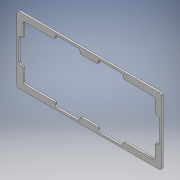
# Autodesk Inventor part: layer3
Saved by Autodesk Inventor 2017 (Build 210142000, 142)
## iProperties
Created: 2021-06-16
Part Number: layer3
Material: Generic
Document SubType Name: Modeling
Designer: Jack
Density: 1 g/cm^3
Appearance: Default
Author: Jack
Autodesk Inventor part; units mm, degrees
ref_plane "YZ Plane" through (0, 0, 0) normal (1, 0, 0) x (0, 1, 0)
ref_plane "XZ Plane" through (0, 0, 0) normal (0, 1, 0) x (-1, 0, 0)
ref_plane "XY Plane" through (0, 0, 0) normal (0, 0, 1) x (1, 0, 0)
sketch "Sketch1" plane through (0, 0, 0) normal (0, 1, 0) x (-1, 0, 0)
  line L0 (-161.0144, 75.423) -> (-161.0144, -74.402)
  line L1 (-156.0144, 80.423) -> (179.5486, 80.423)
  arc A0 (-156.0144, 80.423) -> (-161.0144, 75.423) centre (-156.0144, 75.423) ccw
  arc A1 (-161.0144, -74.402) -> (-156.0144, -79.402) centre (-156.0144, -74.402) ccw
  line L2 (184.5486, -74.402) -> (184.5486, 75.423)
  line L3 (179.5486, -79.402) -> (-156.0144, -79.402)
  arc A2 (179.5486, -79.402) -> (184.5486, -74.402) centre (179.5486, -74.402) ccw
  arc A3 (184.5486, 75.423) -> (179.5486, 80.423) centre (179.5486, 75.423) ccw
  line L4 (-143.0264, 65.4235) -> (-72.3404, 65.4235)
  line L5 (169.5485, 62.4233) -> (169.5485, 33.0083)
  line L6 (-146.0144, -61.402) -> (-146.0144, -31.9917)
  line L7 (-146.0144, 62.4233) -> (-146.0144, 33.0083)
  line L8 (-156.0144, 0.5083) -> (-156.0144, -24.4917)
  line L9 (-156.0144, 0.5083) -> (-156.0144, 25.5083)
  line L10 (-151.0144, -29.4917) -> (-148.5144, -29.4917)
  line L11 (-151.0144, 30.5083) -> (-148.5144, 30.5083)
  line L12 (-7.3404, 65.4235) -> (30.8506, 65.4235)
  line L13 (166.5366, 65.4235) -> (95.8506, 65.4235)
  arc A4 (-151.0144, 30.5083) -> (-156.0144, 25.5083) centre (-151.0144, 25.5083) ccw
  arc A5 (-156.0144, -24.4917) -> (-151.0144, -29.4917) centre (-151.0144, -24.4917) ccw
  arc A6 (-146.0144, -31.9917) -> (-148.5144, -29.4917) centre (-148.5144, -31.9917) ccw
  arc A7 (-148.5144, 30.5083) -> (-146.0144, 33.0083) centre (-148.5144, 33.0083) ccw
  line L14 (179.5485, 0.5083) -> (179.5485, 25.5083)
  line L15 (179.5485, 0.5083) -> (179.5485, -24.4917)
  line L16 (174.5485, 30.5083) -> (172.0485, 30.5083)
  line L17 (174.5485, -29.4917) -> (172.0485, -29.4917)
  arc A8 (174.5485, -29.4917) -> (179.5485, -24.4917) centre (174.5485, -24.4917) ccw
  arc A9 (179.5485, 25.5083) -> (174.5485, 30.5083) centre (174.5485, 25.5083) ccw
  arc A10 (169.5485, 33.0083) -> (172.0485, 30.5083) centre (172.0485, 33.0083) ccw
  arc A11 (172.0485, -29.4917) -> (169.5485, -31.9917) centre (172.0485, -31.9917) ccw
  line L18 (169.5485, -31.9917) -> (169.5485, -61.402)
  line L19 (-39.8404, 75.4235) -> (-64.8404, 75.4235)
  line L20 (-39.8404, 75.4235) -> (-14.8404, 75.4235)
  line L21 (-69.8404, 70.4235) -> (-69.8404, 67.9235)
  line L22 (-9.8404, 70.4235) -> (-9.8404, 67.9235)
  arc A12 (-9.8404, 70.4235) -> (-14.8404, 75.4235) centre (-14.8404, 70.4235) ccw
  arc A13 (-64.8404, 75.4235) -> (-69.8404, 70.4235) centre (-64.8404, 70.4235) ccw
  arc A14 (-72.3404, 65.4235) -> (-69.8404, 67.9235) centre (-72.3404, 67.9235) ccw
  arc A15 (-9.8404, 67.9235) -> (-7.3404, 65.4235) centre (-7.3404, 67.9235) ccw
  line L23 (63.3506, 75.4235) -> (38.3506, 75.4235)
  line L24 (63.3506, 75.4235) -> (88.3506, 75.4235)
  line L25 (33.3506, 70.4235) -> (33.3506, 67.9235)
  line L26 (93.3506, 70.4235) -> (93.3506, 67.9235)
  arc A16 (93.3506, 70.4235) -> (88.3506, 75.4235) centre (88.3506, 70.4235) ccw
  arc A17 (38.3506, 75.4235) -> (33.3506, 70.4235) centre (38.3506, 70.4235) ccw
  arc A18 (30.8506, 65.4235) -> (33.3506, 67.9235) centre (30.8506, 67.9235) ccw
  arc A19 (93.3506, 67.9235) -> (95.8506, 65.4235) centre (95.8506, 67.9235) ccw
  line L27 (166.5485, -64.402) -> (95.8625, -64.402)
  line L28 (-143.0144, -64.402) -> (-72.3284, -64.402)
  line L29 (63.3625, -74.402) -> (88.3625, -74.402)
  line L30 (63.3625, -74.402) -> (38.3625, -74.402)
  line L31 (93.3625, -69.402) -> (93.3625, -66.902)
  line L32 (33.3625, -69.402) -> (33.3625, -66.902)
  arc A20 (33.3625, -69.402) -> (38.3625, -74.402) centre (38.3625, -69.402) ccw
  arc A21 (88.3625, -74.402) -> (93.3625, -69.402) centre (88.3625, -69.402) ccw
  arc A22 (95.8625, -64.402) -> (93.3625, -66.902) centre (95.8625, -66.902) ccw
  arc A23 (33.3625, -66.902) -> (30.8625, -64.402) centre (30.8625, -66.902) ccw
  line L33 (-39.8284, -74.402) -> (-14.8284, -74.402)
  line L34 (-39.8284, -74.402) -> (-64.8284, -74.402)
  line L35 (-9.8284, -69.402) -> (-9.8284, -66.902)
  line L36 (-69.8284, -69.402) -> (-69.8284, -66.902)
  arc A24 (-69.8284, -69.402) -> (-64.8284, -74.402) centre (-64.8284, -69.402) ccw
  arc A25 (-14.8284, -74.402) -> (-9.8284, -69.402) centre (-14.8284, -69.402) ccw
  arc A26 (-7.3284, -64.402) -> (-9.8284, -66.902) centre (-7.3284, -66.902) ccw
  arc A27 (-69.8284, -66.902) -> (-72.3284, -64.402) centre (-72.3284, -66.902) ccw
  line L37 (30.8625, -64.402) -> (-7.3284, -64.402)
  line L38 (-7.3284, -64.402) -> (11.7666, -64.402)
  line L39 (-7.3404, 65.4235) -> (11.7546, 65.4235)
  arc A28 (-143.0144, 65.4235) -> (-146.0144, 62.394) centre (-143.0144, 62.4233) ccw
  arc A29 (169.5485, 62.4233) -> (166.5366, 65.4235) centre (166.6427, 62.5181) ccw
  arc A30 (166.5485, -64.402) -> (169.5485, -61.402) centre (166.5485, -61.402) ccw
  arc A31 (-146.0144, -61.402) -> (-143.0144, -64.402) centre (-143.0144, -61.402) ccw
  point P0 (0, 0)
  constraints: 80 end point, 64 point on circle, 32 centre point, 4 point on line
extrude "Extrusion1" add sketch "Sketch1" along normal blind 4
body "Solid1"
